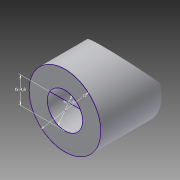
# Autodesk Inventor part: knob
Saved by Autodesk Inventor 2013 (Build 170138000, 138)
## iProperties
Created: 2017-10-13
Part Number: knob
Material: Generic
Document SubType Name: Modeling
Designer: joaquin
Density: 1 g/cm^3
Author: joaquin
Autodesk Inventor part; units mm, degrees
ref_plane "YZ Plane" through (0, 0, 0) normal (1, 0, 0) x (0, 1, 0)
ref_plane "XZ Plane" through (0, 0, 0) normal (0, 1, 0) x (-1, 0, 0)
ref_plane "XY Plane" through (0, 0, 0) normal (0, 0, 1) x (1, 0, 0)
sketch "Sketch1" plane through (0, 0, 0) normal (0, 1, 0) x (-1, 0, 0)
  circle A0 centre (0, 0) radius 3.2
  circle A1 centre (0, 0) radius 6.5
  line L0 (-2.7713, 1.6) -> (2.7713, 1.6)
  dimension "d0" = 6.4
  dimension "d2" = 13
  dimension "d7" = 4.8
  constraints: 2 centre point, 2 coincident, 2 end point, 2 point on circle, 1 horizontal
  measures "d0" diameter of A0
  measures "d2" diameter of A1
extrude "Extrusion1" add sketch "Sketch1" along normal blind 11 contours A0 L0 | L0 A0 | A1
extrude "Extrusion2" cut sketch "Sketch1" along normal blind 2.7 contours A0 L0 | L0 A0
extrude "Extrusion3" cut sketch "Sketch1" along normal blind 9.7 contours A0 L0 picked at (-0.1715, -0.3975)
sketch "Sketch3" plane through (0, 0, 0) normal (1, 0, 0) x (0, 1, 0)
  line L0 (0, 6.5) -> (11, 6.5) projected
  line L1 (11, 6.5) -> (11, -6.5) projected
  line L2 (11, -6.5) -> (0, -6.5) projected
  line L3 (0, -6.5) -> (0, -3.2) projected
  line L4 (0, -3.2) -> (9.7, -3.2) projected
  line L5 (9.7, -3.2) -> (9.7, 1.6) projected
  line L6 (9.7, 1.6) -> (2.7, 1.6) projected
  line L7 (2.7, 1.6) -> (2.7, 3.2) projected
  line L8 (2.7, 3.2) -> (0, 3.2) projected
  line L9 (0, 3.2) -> (0, 6.5) projected
  line L10 (11, 1.9375) -> (7, 6.5)
  point P0 (0, 0)
  dimension "d12" = 1.2
  dimension "d13" = 7
  constraints: 2 end point, 2 point on line
  measures "d12" distance from line of L10 L5.end
  measures "d13" distance of L10.end L0.start
extrude "Extrusion5" cut sketch "Sketch3" along normal through all both and the other way through all contours L0 L1 L10
equation "\"offset\" = 0.2"
body "Solid1"
